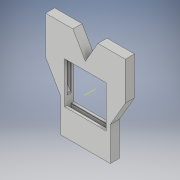
# Autodesk Inventor part: end door
Saved by Autodesk Inventor 2017 (Build 210142000, 142)
## iProperties
Created: 2018-03-09
Part Number: end door
Material: Generic
Document SubType Name: Modeling
Designer: Braxton
Density: 1 g/cm^3
Appearance: Default
Author: Braxton
Autodesk Inventor part; units mm, degrees
ref_plane "YZ Plane" through (0, 0, 0) normal (1, 0, 0) x (0, 1, 0)
ref_plane "XZ Plane" through (0, 0, 0) normal (0, 1, 0) x (-1, 0, 0)
ref_plane "XY Plane" through (0, 0, 0) normal (0, 0, 1) x (1, 0, 0)
sketch "Sketch1" plane through (0, 0, 0) normal (0, 0, 1) x (1, 0, 0)
  line L0 (0, 0) -> (2540, 0)
  line L1 (2540, 0) -> (2540, 2540)
  line L2 (2540, 2540) -> (0, 2540)
  line L3 (0, 2540) -> (0, 0)
  line L4 (-254, 2794) -> (2794, 2794)
  line L5 (2794, 2794) -> (2794, -254)
  line L6 (2794, -254) -> (-254, -254)
  line L7 (-254, -254) -> (-254, 2794)
  line L8 (1270, 0) -> (1270, 1270) construction
  dimension "d0" = 2540
  dimension "d1" = 2540
  dimension "d3" = 254
  dimension "d4" = 254
  dimension "d5" = 254
  dimension "d6" = 254
  dimension "d932" = 1270
  constraints: 18 end point, 4 perpendicular, 2 horizontal, 2 parallel, 1 midpoint, 1 vertical
  measures "d0" distance of L0.start L0.end
  measures "d1" distance of L0.end L1.end
  measures "d3" distance between parallel lines of L2 L4
  measures "d4" distance between parallel lines of L3 L7
  measures "d5" distance between parallel lines of L5 L1
  measures "d6" distance between parallel lines of L6 L0
  measures "d932" distance of L8.start L8.end
extrude "frame" add sketch "Sketch1" along normal mid plane 558.8
ref_plane "middle of part" through (0, 0, 0) normal (0, 0, 1) x (1, 0, 0)
sketch "Sketch8" plane through (0, 0, 0) normal (0, 0, 1) x (1, 0, 0)
  line L0 (2540, 0) -> (0, 0) projected
  line L1 (0, 0) -> (0, -254)
  line L2 (-254, -254) -> (2794, -254) projected
  line L3 (0, -254) -> (2540, -254)
  line L4 (2540, 2540) -> (2540, 0) projected
  line L5 (2540, -254) -> (2540, 0)
  line L6 (2540, 0) -> (0, 0)
  constraints: 8 end point, 3 perpendicular, 1 point on line, 1 vertical
extrude "door slot bottom" cut sketch "Sketch8" along normal mid plane 254
sketch "Sketch7" plane through (0, 0, 0) normal (0, 0, 1) x (1, 0, 0)
  line L0 (102.3298, 595.8453) -> (-251.9439, 1209.4654) construction
  line L1 (-254, -254) -> (-254, 2794) projected
  line L2 (1123.353, 2794) -> (-254, 2794)
  line L3 (-254, 2794) -> (-254, 976.7061)
  line L4 (-254, 976.7061) -> (-50.8, 624.7533)
  line L5 (0, 2540) -> (0, 0) projected
  line L6 (0, 536.7652) -> (0, 2540)
  line L7 (0, 2540) -> (1270, 2540)
  line L8 (1270, 1270) -> (1270, 1044.9425)
  line L9 (1270, 1270) -> (0, 536.7652)
  line L10 (1270, 1620.4707) -> (1270, 1965.6323) construction
  line L11 (1240.6706, 2590.8) -> (1123.353, 2794)
  line L12 (0, 536.7652) -> (-50.8, 536.7652)
  line L13 (-50.8, 536.7652) -> (-50.8, 624.7533)
  line L14 (2437.6702, 595.8453) -> (2791.9439, 1209.4654) construction
  line L15 (2794, -254) -> (2794, 2794)
  line L16 (1416.647, 2794) -> (2794, 2794)
  line L17 (2794, 2794) -> (2794, 976.7061)
  line L18 (2794, 976.7061) -> (2590.8, 624.7533)
  line L19 (2540, 2540) -> (2540, 0)
  line L20 (2540, 536.7652) -> (2540, 2540)
  line L21 (2540, 2540) -> (1270, 2540)
  line L22 (1270, 1270) -> (2540, 536.7652)
  line L23 (1299.3294, 2590.8) -> (1416.647, 2794)
  line L24 (2540, 536.7652) -> (2590.8, 536.7652)
  line L25 (2590.8, 536.7652) -> (2590.8, 624.7533)
  line L26 (1240.6706, 2590.8) -> (1299.3294, 2590.8)
  dimension "d878" = 60
  dimension "d889" = 50.8
  dimension "d901" = 50.8
  constraints: 50 end point, 11 symmetric about line, 4 point on line, 3 perpendicular, 2 horizontal, 2 parallel, 2 vertical, 1 collinear
  measures "d878" angle of L9 L8
  measures "d889" distance of L6.start L12.end
  measures "d901" distance between parallel lines of L7 L26
extrude "top left and right slots" cut sketch "Sketch7" along normal mid plane 254 contours L1 L2 L11 L26 L23 L16 L15 L18 L25 L24 L19 L21 L7 L5 L12 L13 L4
sketch "Sketch12" plane through (0, 0, 0) normal (0, 0, 1) x (1, 0, 0)
  line L0 (0, -25.4) -> (0, -50.8)
  line L1 (0, -254) -> (0, 0) projected
  line L2 (2540, 0) -> (2540, -254) projected
  line L3 (-50.8, 536.7652) -> (-50.8, 2540)
  line L4 (-50.8, 2540) -> (-25.4, 2540)
  line L5 (-25.4, 2540) -> (-25.4, 536.7652)
  line L6 (0, 2540) -> (0, 0) projected
  line L7 (-25.4, 536.7652) -> (-50.8, 536.7652)
  line L8 (0, 2565.4) -> (1270, 2565.4)
  line L9 (2540, 2540) -> (0, 2540) projected
  line L10 (0, 2565.4) -> (0, 2590.8)
  line L11 (0, 2590.8) -> (1270, 2590.8)
  line L12 (1270, 2247.8687) -> (1270, 725.8303) construction
  line L13 (0, -25.4) -> (1270, -25.4)
  line L14 (1270, -50.8) -> (0, -50.8)
  line L15 (2540, -25.4) -> (2540, -50.8)
  line L16 (2590.8, 536.7652) -> (2590.8, 2540)
  line L17 (2590.8, 2540) -> (2565.4, 2540)
  line L18 (2565.4, 2540) -> (2565.4, 536.7652)
  line L19 (2540, 2565.4) -> (1270, 2565.4)
  line L20 (0, 2540) -> (2540, 2540)
  line L21 (2540, 2565.4) -> (2540, 2590.8)
  line L22 (2540, 2590.8) -> (1270, 2590.8)
  line L23 (2540, -25.4) -> (1270, -25.4)
  line L24 (1270, -50.8) -> (2540, -50.8)
  line L25 (2590.8, 536.7652) -> (2540, 536.7652) projected
  line L26 (2565.4, 536.7652) -> (2590.8, 536.7652)
  line L27 (2540, 0) -> (2540, 2540) projected
  dimension "d890" = 25.4
  dimension "d891" = 25.4
  dimension "d893" = 25.4
  dimension "d894" = 25.4
  dimension "d895" = 25.4
  dimension "d902" = 2003.2348
  constraints: 44 end point, 10 symmetric about line, 3 perpendicular, 2 horizontal, 2 vertical, 1 collinear, 1 point on line
  measures "d890" distance between parallel lines of L6 L5
  measures "d891" distance between parallel lines of L5 L3
  measures "d893" distance of L8.start L10.end
  measures "d894" distance from line of L13 L1.end
  measures "d895" distance between parallel lines of L13 L14
  measures "d902" distance of L4.end L5.end
extrude "slots for hiding bars" cut sketch "Sketch12" along normal mid plane 508 contours L13 L23 L2 L24 L14 L0 | L3 L4 L5 L7 | L10 L11 L22 L21 L19 L8 | L25 L18 L17 L16
sketch "Sketch13" plane through (0, 0, 0) normal (0, 0, 1) x (1, 0, 0)
  line L0 (0, -254) -> (0, -50.8) projected
  line L1 (0, -50.8) -> (0, -1346.2)
  line L2 (0, -1346.2) -> (2540, -1346.2)
  line L3 (2540, -50.8) -> (2540, -254) projected
  line L4 (2540, -1346.2) -> (2540, -50.8)
  line L5 (2794, -254) -> (-254, -254) projected
  line L6 (2540, -50.8) -> (0, -50.8) projected
  line L7 (2540, -50.8) -> (0, -50.8)
  line L8 (-50.8, 624.7533) -> (-254, 976.7061) projected
  line L9 (0, 2590.8) -> (1240.6706, 2590.8) projected
  line L10 (507.4358, 4368.8) -> (-1163.2112, 4368.8)
  line L11 (-1163.2112, 4368.8) -> (-1163.2112, 2043.5061)
  line L12 (1270, 3756.6434) -> (1270, 722.7588) construction
  line L13 (2540, 2590.8) -> (1299.3294, 2590.8)
  line L14 (1123.353, 2794) -> (1240.6706, 2590.8) projected
  line L15 (-50.8, 116.7533) -> (-1163.2112, 2043.5061)
  line L16 (-50.8, 624.7533) -> (-909.2112, 2111.5652)
  line L17 (-909.2112, 2111.5652) -> (-909.2112, 4114.8)
  line L18 (-50.8, 536.7652) -> (-50.8, 2540) projected
  line L19 (360.7888, 4114.8) -> (-909.2112, 4114.8)
  line L20 (1240.6706, 2590.8) -> (360.7888, 4114.8)
  line L21 (507.4358, 4368.8) -> (1270, 3048)
  line L22 (0, -50.8) -> (-254, -50.8)
  line L23 (-254, -254) -> (-254, 2794) projected
  line L24 (-254, -50.8) -> (-254, -1600.2)
  line L25 (-254, -1600.2) -> (2794, -1600.2)
  line L26 (2794, -1600.2) -> (2794, -50.8)
  line L27 (2794, 2794) -> (2794, -254) projected
  line L28 (2540, -50.8) -> (2794, -50.8)
  line L29 (1240.6706, 2590.8) -> (1270, 2590.8)
  line L30 (0, 2590.8) -> (2540, 2590.8) projected
  line L31 (1270, 2590.8) -> (1270, 3048)
  line L32 (-50.8, 624.7533) -> (-50.8, 2540) projected
  line L33 (-50.8, 624.7533) -> (-50.8, 116.7533)
  line L34 (2032.5642, 4368.8) -> (3703.2112, 4368.8)
  line L35 (3703.2112, 4368.8) -> (3703.2112, 2043.5061)
  line L36 (1416.647, 2794) -> (1299.3294, 2590.8)
  line L37 (2590.8, 116.7533) -> (3703.2112, 2043.5061)
  line L38 (2590.8, 624.7533) -> (3449.2112, 2111.5652)
  line L39 (3449.2112, 2111.5652) -> (3449.2112, 4114.8)
  line L40 (2179.2112, 4114.8) -> (3449.2112, 4114.8)
  line L41 (1299.3294, 2590.8) -> (2179.2112, 4114.8)
  line L42 (2032.5642, 4368.8) -> (1270, 3048)
  line L43 (1299.3294, 2590.8) -> (1270, 2590.8)
  line L44 (2590.8, 624.7533) -> (2590.8, 116.7533)
  line L45 (2794, 2794) -> (-254, 2794) projected
  point P0 (0, 0)
  dimension "d903" = 1295.4
  dimension "d907" = 254
  dimension "d916" = 254
  dimension "d917" = 254
  dimension "d919" = 254
  dimension "d920" = 254
  dimension "d921" = 254
  dimension "d926" = 655.2112
  dimension "d927" = 1320.8
  constraints: 66 end point, 11 symmetric about line, 6 collinear, 6 perpendicular, 4 parallel, 4 point on line, 4 vertical, 2 horizontal, 1 midpoint
  measures "d903" distance of L0.end L1.end
  measures "d907" distance between parallel lines of L15 L8
  measures "d916" distance between parallel lines of L2 L25
  measures "d917" distance between parallel lines of L26 L4
  measures "d919" distance between parallel lines of L11 L17
  measures "d920" distance between parallel lines of L10 L19
  measures "d921" distance between parallel lines of L21 L20
  measures "d926" distance between parallel lines of L23 L17
  measures "d927" distance between parallel lines of L45 L19
extrude "door recieves" add sketch "Sketch13" along normal mid plane 558.8 contours L1 L2 L4 L5 L26 L25 L24 | L3 L28 L26 L5 | L23 L8 L18 L33 L15 | L15 L11 L10 L21 L31 L45 L20 L19 L17 L16 L23 | L37 L44 L38 L27 | L27 L38 L39 L40 L41 L45 L31 L42 L34 L35 L37 | L45 L31 L29 L14 | L36 L30 L31 L45
sketch "Sketch14" plane through (0, 0, 279.4) normal (0, 0, 1) x (1, 0, 0)
  line L0 (-254, 976.7061) -> (-909.2112, 2111.5652) projected
  line L1 (-909.2112, 2111.5652) -> (-909.2112, 4114.8) projected
  line L2 (-254, 976.7061) -> (-909.2112, 2111.5652)
  line L3 (-909.2112, 2111.5652) -> (-909.2112, 4114.8)
  line L4 (-909.2112, 4114.8) -> (360.7888, 4114.8)
  line L5 (-254, 2794) -> (1123.353, 2794) projected
  line L6 (360.7888, 4114.8) -> (1123.353, 2794)
  line L7 (1123.353, 2794) -> (-254, 2794)
  line L8 (-254, 2794) -> (-254, 976.7061)
  line L9 (3449.2112, 4114.8) -> (2179.2112, 4114.8) projected
  line L10 (1416.647, 2794) -> (2179.2112, 4114.8)
  line L11 (2179.2112, 4114.8) -> (3449.2112, 4114.8)
  line L12 (2794, 976.7061) -> (3449.2112, 2111.5652) projected
  line L13 (3449.2112, 4114.8) -> (3449.2112, 2111.5652)
  line L14 (2794, 2794) -> (2794, 976.7061) projected
  line L15 (3449.2112, 2111.5652) -> (2794, 976.7061)
  line L16 (2794, 976.7061) -> (2794, 2794)
  line L17 (2794, 2794) -> (1416.647, 2794)
  line L18 (2540, -254) -> (0, -254) projected
  line L19 (0, -1346.2) -> (0, -254) projected
  line L20 (0, -254) -> (0, -1346.2)
  line L21 (2540, -1346.2) -> (2540, -254) projected
  line L22 (0, -1346.2) -> (2540, -1346.2)
  line L23 (2540, -1346.2) -> (2540, -254)
  line L24 (2540, -254) -> (0, -254)
  point P0 (0, 0)
  constraints: 32 end point, 6 perpendicular, 5 collinear, 2 parallel, 1 vertical
extrude "front hide door" add sketch "Sketch14" against normal up to surface (152.4 mm away)
sketch "Sketch15" plane through (0, 0, -279.4) normal (0, 0, -1) x (-1, 0, 0)
  line L0 (-1416.647, 2794) -> (-2794, 2794) projected
  line L1 (-3449.2112, 4114.8) -> (-2179.2112, 4114.8) projected
  line L2 (-1416.647, 2794) -> (-2179.2112, 4114.8)
  line L3 (-2179.2112, 4114.8) -> (-3449.2112, 4114.8)
  line L4 (-3449.2112, 2111.5652) -> (-3449.2112, 4114.8) projected
  line L5 (-3449.2112, 4114.8) -> (-3449.2112, 2111.5652)
  line L6 (-3449.2112, 2111.5652) -> (-2794, 976.7061)
  line L7 (-2794, 976.7061) -> (-2794, 2794)
  line L8 (-2794, 2794) -> (-1416.647, 2794)
  line L9 (254, 2794) -> (-1123.353, 2794) projected
  line L10 (-360.7888, 4114.8) -> (909.2112, 4114.8) projected
  line L11 (-1123.353, 2794) -> (-360.7888, 4114.8)
  line L12 (-360.7888, 4114.8) -> (909.2112, 4114.8)
  line L13 (909.2112, 2111.5652) -> (254, 976.7061) projected
  line L14 (909.2112, 4114.8) -> (909.2112, 2111.5652)
  line L15 (909.2112, 2111.5652) -> (254, 976.7061)
  line L16 (254, 976.7061) -> (254, 2794) projected
  line L17 (254, 976.7061) -> (254, 2794)
  line L18 (254, 2794) -> (-1123.353, 2794)
  line L19 (0, -254) -> (0, -1346.2) projected
  line L20 (0, -254) -> (0, -1346.2)
  line L21 (0, -1346.2) -> (-2540, -1346.2) projected
  line L22 (0, -1346.2) -> (-2540, -1346.2)
  line L23 (-2540, -254) -> (0, -254) projected
  line L24 (-2540, -1346.2) -> (-2540, -254)
  line L25 (-2540, -254) -> (0, -254)
  point P0 (0, 0)
  constraints: 32 end point, 6 collinear, 5 perpendicular, 3 parallel
extrude "gap for door pieces" add sketch "Sketch15" against normal up to surface (152.4 mm away)
equation "\"d3\" = d4"
equation "\"d5\" = d4"
equation "\"d6\" = d4"
